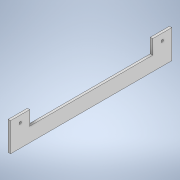
# Autodesk Inventor part: Conveyor Support
Saved by Autodesk Inventor 2022.2 (Build 262287000, 287)
## iProperties
Created: 2022-03-14
Part Number: Conveyor Support
Material: Generic
Document SubType Name: Modeling
Designer: PRASHANTH
Density: 1 g/cm^3
Appearance: Default
Author: PRASHANTH
Autodesk Inventor part; units mm, degrees
ref_plane "YZ Plane" through (0, 0, 0) normal (1, 0, 0) x (0, 1, 0)
ref_plane "XZ Plane" through (0, 0, 0) normal (0, 1, 0) x (-1, 0, 0)
ref_plane "XY Plane" through (0, 0, 0) normal (0, 0, 1) x (1, 0, 0)
sketch "Sketch1" plane through (0, 0, 0) normal (1, 0, 0) x (0, 1, 0)
  line L0 (-30, 168.75) -> (30, 168.75)
  line L1 (30, -168.75) -> (-30, -168.75)
  line L2 (-30, -168.75) -> (-30, 168.75)
  line L3 (30, 168.75) -> (30, 128.75)
  line L4 (0, 128.75) -> (30, 128.75)
  line L5 (30, -168.75) -> (30, -128.75)
  line L6 (0, -128.75) -> (30, -128.75)
  line L7 (30, 168.75) -> (30, 128.75)
  line L8 (30, -128.75) -> (30, -168.75)
  line L9 (0, 128.75) -> (0, -128.75)
  point P0 (0, 0)
  constraints: 20 end point, 5 perpendicular, 3 parallel, 1 horizontal
extrude "Extrusion1" add sketch "Sketch1" along normal blind 5
sketch "Sketch2" plane through (5, 0, 0) normal (1, 0, 0) x (0, 0, -1)
  circle A0 centre (-148.75, 16.0332) radius 2.5
  circle A1 centre (148.6267, 16.0332) radius 2.5
  point P0 (0, 0)
  dimension "d6" = 5
  dimension "d7" = 5
  constraints: 2 centre point
  measures "d6" diameter of A0
  measures "d7" diameter of A1
extrude "Extrusion2" cut sketch "Sketch2" against normal blind 10
body "Solid1"
